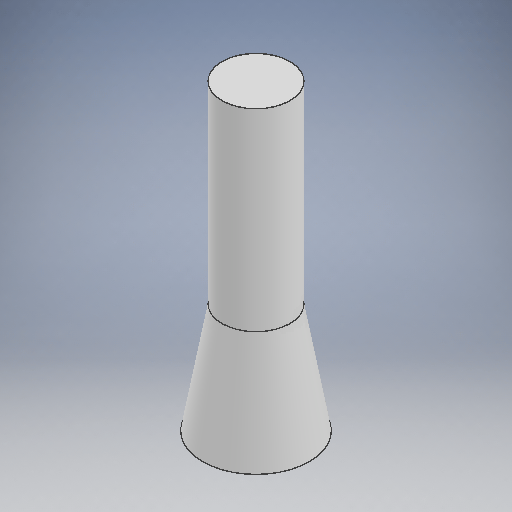
# Autodesk Inventor part: body
Saved by Autodesk Inventor 2025.2 (Build 292293000, 293)
## iProperties
Created: 2025-03-09
Part Number: body
Material: Generic
Document SubType Name: Modeling
Designer: Alex
Density: 1 g/cm^3
Appearance: Default
Author: Alex
Autodesk Inventor part; units mm, degrees
ref_plane "YZ Plane" through (0, 0, 0) normal (1, 0, 0) x (0, 1, 0)
ref_plane "XZ Plane" through (0, 0, 0) normal (0, 1, 0) x (-1, 0, 0)
ref_plane "XY Plane" through (0, 0, 0) normal (0, 0, 1) x (1, 0, 0)
sketch "Sketch1" plane through (0, 0, 0) normal (1, 0, 0) x (0, 1, 0)
  line L0 (0, 0) -> (0, -9.15) construction
  line L1 (0, -9.15) -> (9.0687, -2.8) construction
  line L2 (9.0687, -2.8) -> (9.0687, 0) construction
  line L3 (0, -9.15) -> (0, -29.4542) construction
  line L4 (0, 0) -> (49.8191, 0) construction
  line L5 (9.0687, 0) -> (0, 0)
  line L6 (9.0687, -2.8) -> (25, -2.8)
  line L7 (25, -2.8) -> (25, 0)
  line L8 (25, 0) -> (9.0687, 0)
  line L9 (9.0687, -2.8) -> (0, -4.3991)
  line L10 (0, 0) -> (0, -4.3991)
  dimension "d1" = 125
  dimension "d2" = 5.6
  dimension "d3" = 9.15
  dimension "d5" = 9.0687
  dimension "d6" = 25
  dimension "d8" = 80
  constraints: 22 end point, 3 collinear, 2 horizontal, 2 point on line, 2 vertical, 1 parallel, 1 perpendicular
  measures "d1" angle of L3 L1
  measures "d2" diameter of L1.end L4
  measures "d3" distance of L0.start L0.end
  measures "d5" distance of L0.start L2.end
  measures "d6" distance between parallel lines of L3 L7
  measures "d8" angle of L0 L9
revolve "Revolution1" add sketch "Sketch1" angle 360 about axis through (0, 0, 0) along (0, 1, 0)
body "Solid1"
